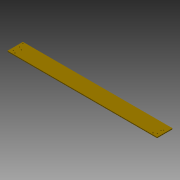
# Autodesk Inventor part: X Rail
Saved by Autodesk Inventor 2013 SP2 (Build 170200200, 200)
## iProperties
Created: 2017-01-25
Part Number: X Rail
Material: Generic
Document SubType Name: Modeling
Designer: Herman de Vries
Density: 1 g/cm^3
Mass: 83.9152 g
Surface Area: 597.165 cm^2
Volume: 83.9152 cm^3
Author: Herman de Vries
Autodesk Inventor part; units mm, degrees
ref_plane "YZ Plane" through (0, 0, 0) normal (1, 0, 0) x (0, 1, 0)
ref_plane "XZ Plane" through (0, 0, 0) normal (0, 1, 0) x (-1, 0, 0)
ref_plane "XY Plane" through (0, 0, 0) normal (0, 0, 1) x (1, 0, 0)
sketch "Sketch1" plane through (0, 0, 0) normal (1, 0, 0) x (0, 1, 0)
  line L0 (0, 0) -> (50, 0)
  line L1 (50, 0) -> (50, 3)
  line L2 (50, 3) -> (0, 3)
  line L3 (0, 3) -> (0, 0)
  dimension "d0" = 50
  dimension "d1" = 3
  constraints: 8 end point, 2 parallel, 1 horizontal, 1 perpendicular
  measures "d0" distance of L2.end L1.end
  measures "d1" distance of L1.end L0.end
extrude "Extrusion1" add sketch "Sketch1" along normal blind 486
sketch "Sketch2" plane through (0, 0, 3) normal (0, 0, 1) x (1, 0, 0)
  circle A0 centre (5.1, 45) radius 1.5
  circle A1 centre (20.1, 25) radius 1.5
  line L0 (0, 0) -> (486, 0) projected
  line L1 (0, 50) -> (486, 50) projected
  line L2 (0, 50) -> (0, 0) projected
  circle A2 centre (481.9, 45) radius 1.5
  line L3 (486, 50) -> (486, 0) projected
  circle A3 centre (462.9, 25) radius 1.5
  circle A4 centre (3, -380) radius 7.5 construction
  line L4 (491.5, -393) -> (472.5, -393) construction
  line L5 (472.5, -393) -> (472.5, 67.7162) construction
  line L6 (472.5, 67.7162) -> (491.5, 67.7162) construction
  line L7 (491.5, 67.7162) -> (491.5, -393) construction
  line L8 (10.5, -380) -> (-4.5, -380) construction
  line L9 (-4.5, -380) -> (-4.5, 66.3205) construction
  line L10 (-4.5, 66.3205) -> (10.5, 66.3205) construction
  line L11 (10.5, 66.3205) -> (10.5, -380) construction
  circle A5 centre (5.1, 45) radius 9.6 construction
  circle A6 centre (20.1, 25) radius 9.6 construction
  circle A7 centre (18.5, 5.5) radius 1.65 projected
  circle A8 centre (9, 30) radius 1.5
  circle A9 centre (9, 10) radius 1.5
  circle A10 centre (477, 10) radius 1.5
  circle A11 centre (477, 30) radius 1.5
  line L12 (469.5, 50) -> (484.5, 50) construction
  line L13 (1.5, 50) -> (16.5, 50) construction
  circle A12 centre (482, -389) radius 9.5 construction
  circle A13 centre (467.5, 5.5) radius 1.65 projected
  point P0 (486, 25)
  point P1 (9, 50)
  point P2 (477, 50)
  dimension "d4" = 3
  dimension "d5" = 3
  dimension "d9" = 3
  dimension "d14" = 20
  dimension "d15" = 5
  dimension "d16" = 3
  dimension "d19" = 5
  dimension "d20" = 20
  dimension "d22" = 9.6
  dimension "d23" = 9.6
  dimension "d24" = 9.6
  dimension "d25" = 9.6
  dimension "d26" = 3
  dimension "d27" = 3
  dimension "d28" = 3
  dimension "d29" = 3
  dimension "d30" = 10
  dimension "d31" = 20
  constraints: 16 end point, 8 centre point, 4 parallel, 4 vertical alignment, 3 horizontal alignment, 3 midpoint, 2 horizontal, 2 perpendicular, 2 tangent, 2 vertical, 1 other
  measures "d4" diameter of A0
  measures "d5" diameter of A1
  measures "d9" diameter of A2
  measures "d14" vertical distance of A1.centre A0.centre
  measures "d15" distance from line of A0.centre L1
  measures "d16" diameter of A3
  measures "d19" distance from line of L1 A2.centre
  measures "d20" vertical distance of A3.centre A2.centre
  measures "d22" distance from line of L9 A0.centre
  measures "d23" distance from line of A1.centre L11
  measures "d24" distance from line of L7 A2.centre
  measures "d25" distance from line of A3.centre L5
  measures "d26" diameter of A8
  measures "d27" diameter of A9
  measures "d28" diameter of A10
  measures "d29" diameter of A11
  measures "d30" distance from line of A9.centre L0
  measures "d31" distance of A9.centre A8.centre
extrude "Extrusion2" cut sketch "Sketch2" against normal blind 10 contours A0 | A1 | A2 | A3 | A7 | A8 | A9 | A10 | A11 | A13
equation "\"d5\" = d4"
equation "\"d9\" = d4"
equation "\"d16\" = d9"
equation "\"d19\" = d15"
equation "\"d20\" = d14"
equation "\"d23\" = d22"
equation "\"d24\" = d22"
equation "\"d25\" = d24"
body "Solid1"
